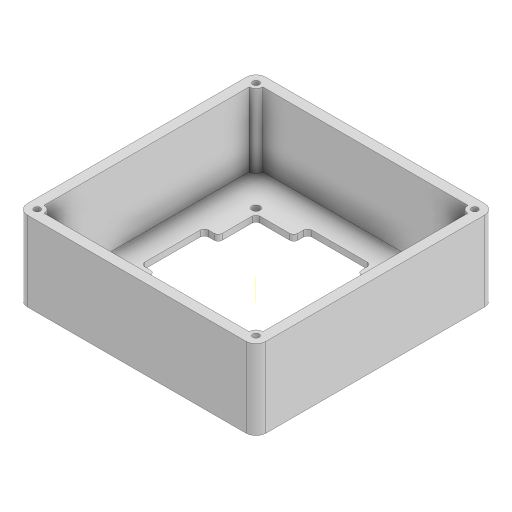
# Autodesk Inventor part: 3D printed box
Saved by Autodesk Inventor 2023 (Build 270158000, 158)
## iProperties
Created: 2022-11-03
Part Number: 3D printed box
Material: Generic
Document SubType Name: Modeling
Designer: ferrerx
Density: 1 g/cm^3
Appearance: Default
Author: ferrerx
Autodesk Inventor part; units mm, degrees
ref_plane "YZ Plane" through (0, 0, 0) normal (1, 0, 0) x (0, 1, 0)
ref_plane "XZ Plane" through (0, 0, 0) normal (0, 1, 0) x (-1, 0, 0)
ref_plane "XY Plane" through (0, 0, 0) normal (0, 0, 1) x (1, 0, 0)
sketch "Sketch1" plane through (0, 0, 0) normal (0, 1, 0) x (-1, 0, 0)
  line L0 (-55, 55) -> (55, 55)
  line L1 (55, 55) -> (55, -55)
  line L2 (55, -55) -> (-55, -55)
  line L3 (-55, -55) -> (-55, 55)
  line L4 (-55, 55) -> (55, -55) construction
  line L5 (55, 55) -> (-55, -55) construction
  line L6 (-12.5, 37.5) -> (12.5, 37.5) construction
  line L7 (12.5, 37.5) -> (12.5, -37.5) construction
  line L8 (12.5, -37.5) -> (-12.5, -37.5) construction
  line L9 (-12.5, -37.5) -> (-12.5, 37.5) construction
  line L10 (-12.5, 37.5) -> (12.5, -37.5) construction
  line L11 (12.5, 37.5) -> (-12.5, -37.5) construction
  line L12 (-37.5, 37.5) -> (37.5, 37.5) construction
  line L13 (37.5, 37.5) -> (37.5, -37.5) construction
  line L14 (37.5, -37.5) -> (-37.5, -37.5) construction
  line L15 (-37.5, -37.5) -> (-37.5, 37.5)
  line L16 (-37.5, 37.5) -> (37.5, -37.5) construction
  line L17 (37.5, 37.5) -> (-37.5, -37.5) construction
  circle A0 centre (37.5, -37.5) radius 2
  circle A1 centre (37.5, 37.5) radius 2
  circle A2 centre (-37.5, 37.5) radius 2
  circle A3 centre (-37.5, -37.5) radius 2
  point P0 (0, 0)
  dimension "d0" = 110
  dimension "d1" = 110
  dimension "d2" = 25
  dimension "d3" = 75
  dimension "d4" = 75
  dimension "d5" = 4
  dimension "d6" = 4
  dimension "d7" = 4
  dimension "d8" = 4
  constraints: 36 end point, 6 midpoint, 6 parallel, 4 centre point, 4 coincident, 3 horizontal, 3 perpendicular, 1 point on line
  measures "d0" distance of L1.end L2.end
  measures "d1" distance of L0.end L1.end
  measures "d2" distance of L7.end L8.end
  measures "d3" distance of L8.end L6.start
  measures "d4" distance of L13.end L14.end
  measures "d5" diameter of A0
  measures "d6" diameter of A1
  measures "d7" diameter of A2
  measures "d8" diameter of A3
extrude "Extrusion1" add sketch "Sketch1" along normal blind 3
sketch "Sketch3" plane through (0, 3, 0) normal (0, 1, 0) x (1, 0, 0)
  line L0 (35, -35) -> (-35, -35)
  line L1 (-35, -35) -> (-35, 35)
  line L2 (-35, 35) -> (35, 35)
  line L3 (35, 35) -> (35, -35)
  line L4 (35, -35) -> (-35, 35) construction
  line L5 (-35, -35) -> (35, 35) construction
  point P0 (0, 0)
  dimension "d18" = 70
  dimension "d19" = 70
  constraints: 12 end point, 2 midpoint, 2 parallel, 1 horizontal, 1 perpendicular
  measures "d18" distance of L1.end L2.end
  measures "d19" distance of L0.end L1.end
extrude "Extrusion3" cut sketch "Sketch3" against normal blind 3
fillet "Fillet1" radius 2 4 edges at (-35, 1.5, 35) (-35, 1.5, -35) (35, 1.5, -35) (35, 1.5, 35)
sketch "Sketch4" plane through (0, 3, 0) normal (0, 1, 0) x (1, 0, 0)
  line L0 (28, -16) -> (42, -16)
  line L1 (42, -16) -> (42, 16)
  line L2 (42, 16) -> (28, 16)
  line L3 (28, 16) -> (28, -16)
  line L4 (28, -16) -> (42, 16) construction
  line L5 (42, -16) -> (28, 16) construction
  line L6 (35, 33) -> (35, -33) projected
  point P0 (0, 0)
  point P1 (35, 0)
  dimension "d23" = 14
  dimension "d24" = 32
  constraints: 12 end point, 3 midpoint, 2 parallel, 1 horizontal, 1 perpendicular
  measures "d23" distance of L1.end L2.end
  measures "d24" distance of L2.end L0.start
extrude "Extrusion4" cut sketch "Sketch4" against normal blind 3
pattern_circular "Circular Pattern2" count 4 over 360 about axis through (0, 0, 0) along (0, 1, 0) of "Extrusion4"
fillet "Fillet2" radius 2 16 edges at (16, 1.5, 35) (-16, 1.5, 35) (16, 1.5, 42) (-16, 1.5, 42) (-35, 1.5, 16) (-42, 1.5, 16) (-42, 1.5, -16) (-35, 1.5, -16) (-16, 1.5, -35) (-16, 1.5, -42) (16, 1.5, -42) (16, 1.5, -35) (35, 1.5, -16) (42, 1.5, -16) (42, 1.5, 16) (35, 1.5, 16)
sketch "Sketch5" plane through (0, 0, 0) normal (0, -1, 0) x (1, 0, 0)
  line L0 (55, -55) -> (-55, -55) projected
  line L1 (-55, 55) -> (55, 55)
  line L2 (55, 55) -> (55, -55)
  line L3 (55, -55) -> (-55, -55)
  line L4 (-55, -55) -> (-55, 55)
  line L5 (-55, 55) -> (55, -55) construction
  line L6 (55, 55) -> (-55, -55) construction
  line L7 (-60, 60) -> (60, 60)
  line L8 (60, 60) -> (60, -60)
  line L9 (60, -60) -> (-60, -60)
  line L10 (-60, -60) -> (-60, 60)
  line L11 (-60, 60) -> (60, -60) construction
  line L12 (60, 60) -> (-60, -60) construction
  point P0 (0, 0)
  dimension "d31" = 5
  constraints: 24 end point, 4 midpoint, 4 parallel, 2 horizontal, 2 perpendicular, 1 point on line
  measures "d31" distance between parallel lines of L0 L9
extrude "Extrusion5" add sketch "Sketch5" against normal blind 40
sketch "Sketch6" plane through (0, 40, 0) normal (0, 1, 0) x (1, 0, 0)
  line L0 (-55, -55) -> (55, -55) projected
  circle A0 centre (-55, -55) radius 3.5
  line L1 (-55, -55) -> (-55, 55) projected
  circle A1 centre (-55, 55) radius 3.5
  line L2 (55, 55) -> (55, -55) projected
  circle A2 centre (55, 55) radius 3.5
  circle A3 centre (55, -55) radius 3.5
  point P0 (0, 0)
  dimension "d34" = 7
  dimension "d35" = 7
  dimension "d36" = 7
  dimension "d37" = 7
  constraints: 4 centre point
  measures "d34" diameter of A2
  measures "d35" diameter of A3
  measures "d36" diameter of A0
  measures "d37" diameter of A1
extrude "Extrusion6" add sketch "Sketch6" against normal up to surface (37 mm away)
sketch "Sketch7" plane through (0, 40, 0) normal (0, 1, 0) x (1, 0, 0)
  arc A0 (55, -51.5) -> (51.5, -55) centre (55, -55) ccw projected
  circle A1 centre (55, -55) radius 1.6
  arc A2 (51.5, 55) -> (55, 51.5) centre (55, 55) ccw projected
  circle A3 centre (55, 55) radius 1.6
  arc A4 (-55, 51.5) -> (-51.5, 55) centre (-55, 55) ccw projected
  circle A5 centre (-55, 55) radius 1.6
  arc A6 (-51.5, -55) -> (-55, -51.5) centre (-55, -55) ccw projected
  circle A7 centre (-55, -55) radius 1.6
  point P0 (0, 0)
  dimension "d40" = 3.2
  dimension "d41" = 3.2
  dimension "d42" = 3.2
  dimension "d43" = 3.2
  constraints: 4 centre point, 4 coincident
  measures "d40" diameter of A7
  measures "d41" diameter of A5
  measures "d42" diameter of A3
  measures "d43" diameter of A1
extrude "Extrusion7" cut sketch "Sketch7" against normal blind 4.5
fillet "Fillet3" radius 5 4 edges at (60, 20, -60) (-60, 20, -60) (60, 20, 60) (-60, 20, 60)
body "Solid1"
